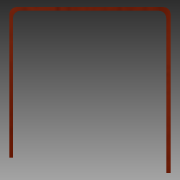
# Autodesk Inventor part: back-cover
Saved by Autodesk Inventor 2015 (Build 190159000, 159)
## iProperties
Created: 2014-07-15
Part Number: back-cover
Material: Wood (Oak)
Document SubType Name: Modeling
Designer: pc
Density: 0.76 g/cm^3
Appearance: White Oak - Natural Medium Gloss
d56: 42.000 mm
wallw: 42.000 mm
wall1_thick: 8.000 mm
wall2_thick: 6.400 mm
wall3_thick: 4.000 mm
wall1slot: 8.120 mm
wall2slot: 6.520 mm
wall3slot: 4.120 mm
gap1: 30.000 mm
gap2: 28.000 mm
baseh: 79.120 mm
basew: 44.000 mm
base_thick: 6.000 mm
base_slots_depth: 4.000 mm
d57: 40.000 mm
printer3dtolerance: 0.120 mm
wallh: 44.000 mm
cornerrad: 2.000 mm
baseextra: 2.000 mm
Author: pc
Autodesk Inventor part; units mm, degrees
ref_plane "YZ Plane" through (0, 0, 0) normal (1, 0, 0) x (0, 1, 0)
ref_plane "XZ Plane" through (0, 0, 0) normal (0, 1, 0) x (-1, 0, 0)
ref_plane "XY Plane" through (0, 0, 0) normal (0, 0, 1) x (1, 0, 0)
sketch "Base" plane through (0, 0, 0) normal (0, 0, 1) x (1, 0, 0)
  line L0 (21.937, -23.2024) -> (21.937, 20.9976)
  line L1 (21.937, 20.9976) -> (-19.8525, 20.9976)
  line L2 (-19.8525, 20.9976) -> (-19.8525, -19.0024)
  line L3 (-19.8525, -19.0024) -> (21.937, 20.9976) construction
  line L4 (21.937, -23.2024) -> (-19.8525, 20.9976) construction
  line L5 (23.1576, -23.2024) -> (23.1576, 21.9976)
  line L6 (23.1576, 21.9976) -> (-20.8525, 21.9976)
  line L7 (-20.8525, 21.9976) -> (-20.8525, 20.9976)
  line L8 (-20.8525, 20.9976) -> (-20.8525, -19.0024)
  line L9 (-19.8525, -19.0024) -> (-20.8525, -19.0024)
  line L10 (21.937, -23.2024) -> (23.1576, -23.2024)
  point P0 (0, 0)
  dimension "d56" = 42
  dimension "d57" = 40
  dimension "d92" = 1
  dimension "d95" = 1
  constraints: 22 end point, 4 parallel, 3 horizontal, 3 point on line, 1 vertical
  measures "d56" distance of L2.end L0.start
  measures "d57" distance of L1.end L2.end
  measures "d92" distance between parallel lines of L2 L7
  measures "d95" distance between parallel lines of L1 L6
extrude "Extrusion8" add sketch "Base" along normal blind 44.4
fillet "Fillet5" radius 2 1 edges at (-19.8525, 20.9976, 22.2)
fillet "Fillet6" radius 2 1 edges at (21.937, 20.9976, 22.2)
fillet "Fillet7" radius 2 1 edges at (-20.8525, 21.9976, 22.2)
fillet "Fillet8" radius 2 1 edges at (23.1576, 21.9976, 22.2)
equation "\"d56\" = wallw"
equation "\"d57\" = wallh - base_slots_depth"
equation "\"d92\" = 0.5 * baseextra"
equation "\"d95\" = d92"
equation "\"d93\" = wall1_thick + gap1 + wall2_thick"
equation "\"d96\" = cornerrad"
equation "\"d97\" = cornerrad"
equation "\"d98\" = cornerrad"
equation "\"d99\" = cornerrad"
equation "\"printer3dtolerance\" = 0.12"
equation "\"wallw\" = 42"
equation "\"wallh\" = 44"
equation "\"cornerrad\" = 2"
equation "\"baseextra\" = 2"
equation "\"wall1_thick\" = 8"
equation "\"wall2_thick\" = 6.4"
equation "\"wall3_thick\" = 4"
equation "\"wall1slot\" = 8.12"
equation "\"wall2slot\" = 6.52"
equation "\"wall3slot\" = 4.12"
equation "\"gap1\" = 30"
equation "\"gap2\" = 28"
equation "\"baseh\" = 79.12"
equation "\"basew\" = 44"
equation "\"base_thick\" = 6"
equation "\"base_slots_depth\" = 4"
equation "\"d26\" = 8.12"
equation "\"d27\" = 42"
equation "\"d28\" = 44"
equation "\"d29\" = 28"
equation "\"d31\" = 4.12"
equation "\"d32\" = 6.52"
equation "\"d33\" = 79.12"
equation "\"d39\" = 8.12"
equation "\"d40\" = 42"
equation "\"d41\" = 44"
equation "\"d48\" = 8.12"
equation "\"d49\" = 42"
equation "\"d50\" = 8.12"
equation "\"d51\" = 42"
equation "\"d52\" = 44"
equation "\"d53\" = 44"
equation "\"d71\" = 8.12"
equation "\"d72\" = 42"
equation "\"d73\" = 2"
equation "\"d74\" = 44"
equation "\"distancefrombottom\" = 34"
equation "\"servosmallcircledia\" = 5.92"
equation "\"servo9gw\" = 22.8"
equation "\"servomountsquare\" = 6"
equation "\"servopolygonl\" = 5.92"
equation "\"servopolygonr\" = 6.12"
equation "\"distancefromleft\" = 26"
equation "\"servobigcircledia\" = 11.62"
equation "\"servomounth\" = 4"
equation "\"wall3slotd\" = 2"
equation "\"wall3slotw\" = 36"
equation "\"adapterh\" = 16"
equation "\"adapterw\" = 32"
equation "\"wall3slotd_1\" = 2"
body "Solid3"
